PLATE_LV_BOTTOM (Autodesk Fusion 360 design; units mm, degrees)
Autodesk Fusion 360 part; units mm, degrees
note: some values were not read from the file. Set by a fixed rule: which sketch regions a step uses.
sketch "Esquisse1" plane through (0, 0, 0) normal (0, 0, 1) x (1, 0, 0)
  line L0 (100, 78) -> (-100, 78)
  line L1 (-100, 78) -> (-100, -78)
  line L2 (-100, -78) -> (100, -78)
  line L3 (100, -78) -> (100, 78)
  line L4 (100, 78) -> (-100, -78) construction
  line L5 (-100, 78) -> (100, -78) construction
  line L6 (103, -75) -> (-103, -75)
  line L7 (-103, -75) -> (-103, 75)
  line L8 (-103, 75) -> (103, 75)
  line L9 (103, 75) -> (103, -75)
  line L10 (103, -75) -> (-103, 75) construction
  line L11 (-103, -75) -> (103, 75) construction
  dimension "d1" = 200
  dimension "d2" = 206
  dimension "d3" = 150
  dimension "d4" = 156
  constraint horizontal L0
  constraint perpendicular L0 L1
  constraint parallel L0 L2
  constraint parallel L1 L3
  constraint coincident L4 origin
  constraint coincident L5 origin
  constraint horizontal L6
  constraint perpendicular L6 L7
  constraint parallel L6 L8
  constraint parallel L7 L9
  constraint coincident L10 origin
  constraint coincident L11 origin
  measures "d1" distance of L0.start L0.end
  measures "d2" distance of L7.end L8.end
  measures "d3" distance of L6.end L7.end
  measures "d4" distance of L0.end L1.end
extrude "Extrusion1" add sketch "Esquisse1" along normal blind 3
sketch "Esquisse3" plane through (0, 0, 3) normal (0, 0, 1) x (-1, 0, 0)
  line L0 (-100, -75) -> (-100, -78)
  line L1 (-100, -78) -> (100, -78)
  line L2 (100, -78) -> (100, -75)
  line L3 (100, -75) -> (103, -75)
  line L4 (103, -75) -> (103, 75)
  line L5 (103, 75) -> (100, 75)
  line L6 (100, 75) -> (100, 78)
  line L7 (100, 78) -> (-100, 78)
  line L8 (-100, 78) -> (-100, 75)
  line L9 (-100, 75) -> (-103, 75)
  line L10 (-103, 75) -> (-103, -75)
  line L11 (-103, -75) -> (-100, -75)
  line L12 (-63.5, 31.75) -> (63.5, 31.75)
  line L13 (63.5, 31.75) -> (63.5, -31.75)
  line L14 (63.5, -31.75) -> (-63.5, -31.75)
  line L15 (-63.5, -31.75) -> (-63.5, 31.75)
  line L16 (-63.5, 31.75) -> (63.5, -31.75) construction
  line L17 (63.5, 31.75) -> (-63.5, -31.75) construction
  circle A0 centre (63.5, -31.75) radius 1.6
  circle A1 centre (63.5, 31.75) radius 1.6
  circle A2 centre (-63.5, -31.75) radius 1.6
  circle A3 centre (-63.5, 31.75) radius 1.6
  dimension "d18" = 63.5
  dimension "d19" = 127
  dimension "d20" = 3.2
  dimension "d21" = 3.2
  dimension "d22" = 3.2
  dimension "d23" = 3.2
  constraint horizontal L12
  constraint perpendicular L12 L13
  constraint parallel L12 L14
  constraint parallel L13 L15
  constraint coincident L16 origin
  constraint coincident L17 origin
  constraint coincident L13.end L14.start
  constraint coincident L12.end L13.start
  constraint coincident L14.end L15.start
  constraint coincident L12.start L15.end
  measures "d18" distance of L12.start L14.end
  measures "d19" distance of L13.end L14.end
  measures "d20" diameter of A0
  measures "d21" diameter of A1
  measures "d22" diameter of A2
  measures "d23" diameter of A3
extrude "Extrusion3" cut sketch "Esquisse3" against normal blind 3 contours L12 L15 A3 | L12 L15 A3 | L12 L13 A1 | L12 L13 A1 | L14 L15 A2 | L14 L15 A2 | L13 L14 A0 | L13 L14 A0
equation "d2 = d1 + ( 2 * 3 ) * 1 mm"
equation "d4 = d3 + ( 2 * 3 ) * 1 mm"
